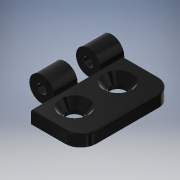
# Autodesk Inventor part: Charnière A
Saved by Autodesk Inventor 2017 (Build 210142000, 142)
## iProperties
Company: FABLAB Frenchmakers
Part Number: Charnière A
Material: Plastique ABS
Document SubType Name: Modeling
Designer: FABLAB Frenchmakers
Density: 1.06 g/cm^3
Appearance: Lisse - Noir
Project: 1400-PopCorn Machine
Catalog Web Link: http://frenchmakers.com/
Stock Number: 1400-05-01
Author: Adrien MARY
Autodesk Inventor part; units mm, degrees
ref_plane "YZ Plane" through (0, 0, 0) normal (1, 0, 0) x (0, 1, 0)
ref_plane "XZ Plane" through (0, 0, 0) normal (0, 1, 0) x (-1, 0, 0)
ref_plane "XY Plane" through (0, 0, 0) normal (0, 0, 1) x (1, 0, 0)
sketch "Esquisse7" plane through (0, 0, 0) normal (0, 0, 1) x (1, 0, 0)
  line L0 (0, -15) -> (16, -15)
  line L1 (16, -15) -> (16, 15)
  line L2 (16, 15) -> (0, 15)
  line L3 (0, 15) -> (0, -15)
  point P0 (0, 0)
  point P1 (0, 0)
  dimension "Largueur" = 16
  dimension "Hauteur" = 30
  constraints: 8 end point, 2 parallel, 1 coincident, 1 horizontal, 1 midpoint, 1 perpendicular
  measures "Largueur" distance of L1.end L2.end
  measures "Hauteur" distance of L0.end L1.end
extrude "Extrusion4" add sketch "Esquisse7" along normal blind 3.8
sketch "Esquisse9" plane through (0, 15, 0) normal (0, 1, 0) x (1, 0, 0)
  arc A0 (-4, 0) -> (0, -4) centre (-4, -4) ccw
  line L0 (0, 0) -> (0, -3.8) construction
  line L1 (16, 0) -> (0, 0) construction
  line L2 (-4, 0) -> (0, 0)
  line L3 (0, 0) -> (0, -4)
  dimension "d41" = 8
  constraints: 4 end point, 4 tangent, 2 collinear, 2 point on circle, 1 centre point
  measures "d41" diameter of A0
extrude "Extrusion6" add sketch "Esquisse9" against normal blind 7.5
pattern_linear "Réseau rectangulaire3" count 2 spacing 15 along (0, -1, 0) of "Extrusion6"
sketch "Esquisse10" plane through (16, 15, 3.8) normal (0, 1, 0) x (1, 0, 0)
  arc A0 (-20, 3.8) -> (-16, -0.2) centre (-20, -0.2) ccw construction
  point P0 (-16, 3.8)
  point P1 (-16.0515, -0.84)
  constraints: 1 coincident
hole "Perçage2" at (-4, 15, 4) direction (0, -1, 0) diameter 3 end through all
fillet "Congé4" radius 5 2 edges at (16, 15, 1.9) (16, -15, 1.9)
sketch "Esquisse11" plane through (0, 0, 3.8) normal (0, 0, 1) x (1, 0, 0)
  line L0 (11, 15) -> (0, 15) construction
  point P0 (0, 0)
  point P1 (5.9678, 7)
  point P2 (5.9678, -7)
  point P3 (0.9356, 15)
  point P4 (5.9678, 15)
  dimension "d56" = 14
  dimension "d57" = 7
  constraints: 2 vertical alignment, 1 point on line
  measures "d56" distance of point (5.968, 7) point (5.968, -7)
  measures "d57" vertical distance of point (5.968, 7) point (0, 0)
hole "Perçage3" at (5.9678, 7, 3.8) at (5.9678, -7, 3.8) direction (0, 0, -1) diameter 5 end through all countersink diameter 9 countersink angle 75
fillet "Congé5" radius 0.5 5 edges at (14.5355, 13.5355, 3.8) (16, 0, 3.8) (14.5355, -13.5355, 3.8) (5.5, -15, 3.8) (5.5, 15, 3.8)
equation "\"d42\" = 0.25 * Hauteur"
equation "\"d47\" = 0.5 * Hauteur"
equation "\"d57\" = 0.5 * d56"
equation "\"pi\" = 3.141593"
equation "\"nombredor\" = 1.61803"
